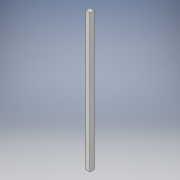
# Autodesk Inventor part: Barre
Saved by Autodesk Inventor 2019 (Build 230136000, 136)
## iProperties
Created: 2020-03-11
Part Number: Barre
Material: Générique
Document SubType Name: Modeling
Designer: Quentin
Density: 1 g/cm^3
Appearance: Par défaut
Author: Quentin
Autodesk Inventor part; units mm, degrees
ref_plane "YZ Plane" through (0, 0, 0) normal (1, 0, 0) x (0, 1, 0)
ref_plane "XZ Plane" through (0, 0, 0) normal (0, 1, 0) x (-1, 0, 0)
ref_plane "XY Plane" through (0, 0, 0) normal (0, 0, 1) x (1, 0, 0)
sketch "Esquisse1" plane through (0, 0, 0) normal (0, 0, 1) x (1, 0, 0)
  line L0 (0, 0) -> (0, 155)
  line L1 (0, 0) -> (5, 0)
  line L2 (5, 0) -> (5, 155)
  line L3 (5, 155) -> (0, 155)
  dimension "d0" = 155
  dimension "d1" = 5
  constraints: 8 end point, 2 perpendicular, 1 horizontal, 1 vertical
  measures "d0" distance of L0.start L0.end
  measures "d1" distance of L0.start L1.end
extrude "Extrusion1" add sketch "Esquisse1" along normal blind 5
